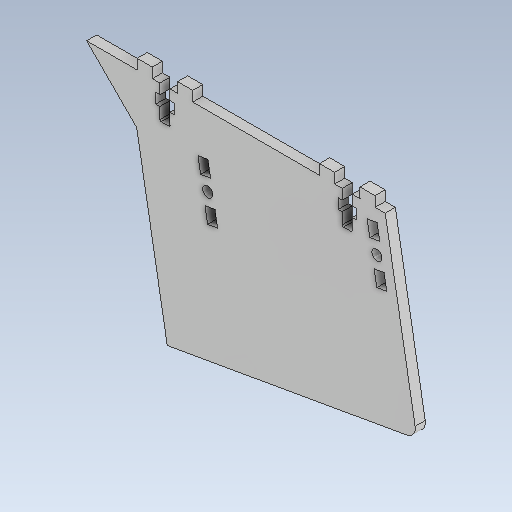
# Autodesk Inventor part: tc_support_front
Saved by Autodesk Inventor 2020.1 (Build 241239000, 239)
## iProperties
Created: 2019-07-16
Part Number: tc_support_front
Material: Acier inoxydable
Document SubType Name: Modeling
Designer: Thibault
Density: 8 g/cm^3
Appearance: Semi-poli
Author: Thibault
Autodesk Inventor part; units mm, degrees
ref_plane "YZ Plane" through (0, 0, 0) normal (1, 0, 0) x (0, 1, 0)
ref_plane "XZ Plane" through (0, 0, 0) normal (0, 1, 0) x (-1, 0, 0)
ref_plane "XY Plane" through (0, 0, 0) normal (0, 0, 1) x (1, 0, 0)
sketch "Anchor (screw side)" plane through (0, 0, 0) normal (0, 0, 1) x (1, 0, 0)
  circle A0 centre (93.7814, 50.2592) radius 1
  line L0 (91.2814, 51.2592) -> (88.2814, 51.2592)
  line L1 (88.2814, 51.2592) -> (88.2814, 49.2592)
  line L2 (88.2814, 49.2592) -> (91.2814, 49.2592)
  line L3 (91.2814, 49.2592) -> (91.2814, 51.2592)
  line L4 (99.2814, 51.2592) -> (96.2814, 51.2592)
  line L5 (96.2814, 51.2592) -> (96.2814, 49.2592)
  line L6 (96.2814, 49.2592) -> (99.2814, 49.2592)
  line L7 (99.2814, 49.2592) -> (99.2814, 51.2592)
  line L8 (91.2814, 51.2592) -> (96.2814, 49.2592) construction
  line L9 (96.2814, 51.2592) -> (91.2814, 49.2592) construction
  line L10 (86.2814, 53.2592) -> (101.2814, 53.2592) construction
  line L11 (101.2814, 53.2592) -> (101.2814, 47.2592) construction
  line L12 (101.2814, 47.2592) -> (86.2814, 47.2592) construction
  line L13 (86.2814, 47.2592) -> (86.2814, 53.2592) construction
  point P0 (103.5798, 50.1132)
  dimension "d27" = 2
  dimension "d28" = 3
  dimension "d29" = 2
  dimension "d30" = 3
  dimension "d32" = 5
  dimension "d34" = 2
  dimension "d35_1" = 2
  dimension "d36_1" = 2
  dimension "d37" = 2
  measures "d27" diameter of A0
  measures "d28" distance of L2.end L1.end
  measures "d29" distance of L1.end L0.end
  measures "d30" distance of L6.end L5.end
  measures "d32" distance between parallel lines of L5 L3
  measures "d34" distance between parallel lines of L0 L10
  measures "d35_1" distance between parallel lines of L12 L2
  measures "d36_1" distance between parallel lines of L11 L7
  measures "d37" distance between parallel lines of L13 L1
sketch "Anchor (nut side)" plane through (0, 0, 0) normal (0, 0, 1) x (1, 0, 0)
  line L0 (10, 0) -> (8.5, 0)
  line L1 (8.5, 0) -> (8.5, -2)
  line L2 (8.5, -2) -> (9.3, -2)
  line L3 (9.3, -2) -> (9.3, -4)
  line L4 (5.7, -4) -> (5.7, -2)
  line L5 (5.7, -2) -> (6.5, -2)
  line L6 (6.5, -2) -> (6.5, 0)
  line L7 (6.5, 0) -> (5, 0)
  line L8 (2, 0) -> (2, 2)
  line L9 (2, 0) -> (3, 0) construction
  line L10 (2, 2) -> (5, 2)
  line L11 (5, 2) -> (5, 0)
  line L12 (5, 2) -> (7, 2) construction
  line L13 (10, 0) -> (10, 2)
  line L14 (10, 2) -> (13, 2)
  line L15 (13, 2) -> (13, 0)
  line L16 (0, 0) -> (2, 0)
  line L17 (13, 0) -> (15, 0)
  line L18 (5.7, -4) -> (6.5, -4)
  line L19 (9.3, -4) -> (8.5, -4)
  line L20 (6.5, -4) -> (6.5, -6.25)
  line L21 (8.5, -4) -> (8.5, -6.25)
  line L22 (6.75, -6.5) -> (7.5, -6.5)
  arc A0 (6.5, -6.25) -> (6.75, -6.5) centre (6.75, -6.25) ccw
  arc A1 (8.25, -6.5) -> (8.5, -6.25) centre (8.25, -6.25) ccw
  line L23 (7.5, -7.2938) -> (7.5, -4.9797)
  line L24 (7.5, -6.5) -> (8.25, -6.5)
  point P0 (9.1321, -0.6227)
  point P1 (6.5, -6.5)
  point P2 (8.5, -6.5)
  dimension "d3" = 2
  dimension "d7" = 5
  dimension "d10" = 1.5
  dimension "d11" = 2
  dimension "d12" = 0.8
  dimension "d13" = 2
  dimension "d14" = 0.8
  dimension "d15" = 2
  dimension "d18" = 2
  dimension "d19" = 0.8
  dimension "d20" = 0.8
  dimension "d21" = 2.5
  dimension "d22" = 2.5
  dimension "d23" = 2
  dimension "d38" = 2
  dimension "d39" = 0.25
  dimension "d118" = 2
  dimension "d120" = 3
  measures "d3" distance of L16.start L8.start
  measures "d7" distance of L7.end L0.start
  measures "d10" distance of L0.start L0.end
  measures "d11" distance of L0.end L1.end
  measures "d12" distance of L1.end L2.end
  measures "d13" distance of L2.end L3.end
  measures "d14" distance of L4.end L5.end
  measures "d15" distance of L6.end L0.end
  measures "d18" distance of L15.end L17.end
  measures "d19" distance of L4.start L18.end
  measures "d20" distance of L3.end L19.end
  measures "d21" distance of L18.end point (6.5, -6.5)
  measures "d22" distance of L19.end point (8.5, -6.5)
  measures "d23" distance of L18.end L19.end
  measures "d38" distance between parallel lines of L16 L10
  measures "d39" radius of A0
  measures "d118" distance between parallel lines of L0 L14
  measures "d120" distance of L8.end L10.end
derived "shared_parameters.ipt"
sketch "Esquisse1" plane through (0, 0, 0) normal (0, 0, 1) x (1, 0, 0)
  line L0 (-2.1192, 7.2641) -> (18.9808, 7.2641)
  line L1 (-17.1192, 7.2641) -> (-25.1192, 7.2641)
  line L2 (-25.1192, 7.2641) -> (-15.2156, -2.6395)
  line L3 (39.9012, -26.3124) -> (33.9808, 7.2641)
  line L4 (38.2789, -28.6293) -> (-9.1581, -36.9937)
  line L5 (-2.0657, -1.8526) -> (7.9343, -1.7975) construction
  arc A0 (38.2789, -28.6293) -> (39.9012, -26.3124) centre (37.9316, -26.6596) ccw
  line L6 (-9.1581, -36.9937) -> (-15.2156, -2.6395)
  line L7 (-7.1192, 7.2641) -> (-8.6192, 7.2641)
  line L8 (-8.6192, 7.2641) -> (-8.6192, 5.2641)
  line L9 (-8.6192, 5.2641) -> (-7.8192, 5.2641)
  line L10 (-7.8192, 5.2641) -> (-7.8192, 3.2641)
  line L11 (-11.4192, 3.2641) -> (-11.4192, 5.2641)
  line L12 (-11.4192, 5.2641) -> (-10.6192, 5.2641)
  line L13 (-10.6192, 5.2641) -> (-10.6192, 7.2641)
  line L14 (-10.6192, 7.2641) -> (-12.1192, 7.2641)
  line L15 (-15.1192, 7.2641) -> (-15.1192, 9.2641)
  line L16 (-15.1192, 7.2641) -> (-14.1192, 7.2641) construction
  line L17 (-15.1192, 9.2641) -> (-12.1192, 9.2641)
  line L18 (-12.1192, 9.2641) -> (-12.1192, 7.2641)
  line L19 (-12.1192, 9.2641) -> (-10.1192, 9.2641) construction
  line L20 (-7.1192, 7.2641) -> (-7.1192, 9.2641)
  line L21 (-7.1192, 9.2641) -> (-4.1192, 9.2641)
  line L22 (-4.1192, 9.2641) -> (-4.1192, 7.2641)
  line L23 (-17.1192, 7.2641) -> (-15.1192, 7.2641)
  line L24 (-4.1192, 7.2641) -> (-2.1192, 7.2641)
  line L25 (-11.4192, 3.2641) -> (-10.6192, 3.2641)
  line L26 (-7.8192, 3.2641) -> (-8.6192, 3.2641)
  line L27 (-10.6192, 3.2641) -> (-10.6192, 1.0141)
  line L28 (-8.6192, 3.2641) -> (-8.6192, 1.0141)
  line L29 (-10.3692, 0.7641) -> (-9.6192, 0.7641)
  arc A1 (-10.6192, 1.0141) -> (-10.3692, 0.7641) centre (-10.3692, 1.0141) ccw
  arc A2 (-8.8692, 0.7641) -> (-8.6192, 1.0141) centre (-8.8692, 1.0141) ccw
  line L30 (-9.6192, -0.0297) -> (-9.6192, 2.2844)
  line L31 (-9.6192, 0.7641) -> (-8.8692, 0.7641)
  line L32 (28.9808, 7.2641) -> (27.4808, 7.2641)
  line L33 (27.4808, 7.2641) -> (27.4808, 5.2641)
  line L34 (27.4808, 5.2641) -> (28.2808, 5.2641)
  line L35 (28.2808, 5.2641) -> (28.2808, 3.2641)
  line L36 (24.6808, 3.2641) -> (24.6808, 5.2641)
  line L37 (24.6808, 5.2641) -> (25.4808, 5.2641)
  line L38 (25.4808, 5.2641) -> (25.4808, 7.2641)
  line L39 (25.4808, 7.2641) -> (23.9808, 7.2641)
  line L40 (20.9808, 7.2641) -> (20.9808, 9.2641)
  line L41 (20.9808, 7.2641) -> (21.9808, 7.2641) construction
  line L42 (20.9808, 9.2641) -> (23.9808, 9.2641)
  line L43 (23.9808, 9.2641) -> (23.9808, 7.2641)
  line L44 (23.9808, 9.2641) -> (25.9808, 9.2641) construction
  line L45 (28.9808, 7.2641) -> (28.9808, 9.2641)
  line L46 (28.9808, 9.2641) -> (31.9808, 9.2641)
  line L47 (31.9808, 9.2641) -> (31.9808, 7.2641)
  line L48 (18.9808, 7.2641) -> (20.9808, 7.2641)
  line L49 (31.9808, 7.2641) -> (33.9808, 7.2641)
  line L50 (24.6808, 3.2641) -> (25.4808, 3.2641)
  line L51 (28.2808, 3.2641) -> (27.4808, 3.2641)
  line L52 (25.4808, 3.2641) -> (25.4808, 1.0141)
  line L53 (27.4808, 3.2641) -> (27.4808, 1.0141)
  line L54 (25.7308, 0.7641) -> (26.4808, 0.7641)
  arc A3 (25.4808, 1.0141) -> (25.7308, 0.7641) centre (25.7308, 1.0141) ccw
  arc A4 (27.2308, 0.7641) -> (27.4808, 1.0141) centre (27.2308, 1.0141) ccw
  line L55 (26.4808, -0.0297) -> (26.4808, 2.2844)
  line L56 (26.4808, 0.7641) -> (27.2308, 0.7641)
  circle A5 centre (32.3451, -0.7359) radius 1
  line L57 (31.7944, -3.3716) -> (32.3154, -6.326)
  line L58 (32.3154, -6.326) -> (34.285, -5.9787)
  line L59 (34.285, -5.9787) -> (33.764, -3.0243)
  line L60 (33.764, -3.0243) -> (31.7944, -3.3716)
  line L61 (30.4052, 4.5069) -> (30.9262, 1.5525)
  line L62 (30.9262, 1.5525) -> (32.8958, 1.8998)
  line L63 (32.8958, 1.8998) -> (32.3748, 4.8542)
  line L64 (32.3748, 4.8542) -> (30.4052, 4.5069)
  line L65 (31.7944, -3.3716) -> (32.8958, 1.8998) construction
  line L66 (30.9262, 1.5525) -> (33.764, -3.0243) construction
  line L67 (30.693, -8.6429) -> (28.0883, 6.1292) construction
  line L68 (28.0883, 6.1292) -> (33.9972, 7.1711) construction
  line L69 (33.9972, 7.1711) -> (36.6019, -7.601) construction
  line L70 (36.6019, -7.601) -> (30.693, -8.6429) construction
  circle A6 centre (-1.1384, -6.6399) radius 1
  line L71 (-0.5877, -4.0043) -> (-1.1086, -1.0498)
  line L72 (-1.1086, -1.0498) -> (-3.0782, -1.3971)
  line L73 (-3.0782, -1.3971) -> (-2.5573, -4.3516)
  line L74 (-2.5573, -4.3516) -> (-0.5877, -4.0043)
  line L75 (0.8015, -11.8827) -> (0.2806, -8.9283)
  line L76 (0.2806, -8.9283) -> (-1.6891, -9.2756)
  line L77 (-1.6891, -9.2756) -> (-1.1681, -12.23)
  line L78 (-1.1681, -12.23) -> (0.8015, -11.8827)
  line L79 (-0.5877, -4.0043) -> (-1.6891, -9.2756) construction
  line L80 (0.2806, -8.9283) -> (-2.5573, -4.3516) construction
  line L81 (0.5137, 1.2671) -> (3.1184, -13.505) construction
  line L82 (3.1184, -13.505) -> (-2.7904, -14.5469) construction
  line L83 (-2.7904, -14.5469) -> (-5.3952, 0.2252) construction
  line L84 (-5.3952, 0.2252) -> (0.5137, 1.2671) construction
  point P0 (40.2485, -28.282)
  point P1 (22.4992, -2.0098)
  point P2 (32.3451, -0.7359)
  point P3 (-1.1384, -6.6399)
  point P4 (33.9808, 7.2641)
  dimension "d33" = 59.1
  dimension "d44" = 23
  dimension "d46" = 2
  dimension "d49" = 10
  dimension "d52" = 2
  dimension "d53" = 36
  dimension "d54" = 8
  dimension "d57" = 45
  dimension "d58" = 10
  constraints: 14 end point, 3 horizontal, 2 point on circle, 2 point on line, 2 tangent, 1 centre point, 1 parallel, 1 perpendicular, 6 other
  measures "d33" distance of L3.end L1.end
  measures "d46" radius of A0
  measures "d57" angle of L2 L1
  measures "d58" angle of L4 L0
extrude "Extrusion1" add sketch "Esquisse1" along normal blind 2
derived "tc_base_plate.ipt"
equation "\"d33\" = tc_base_width"
equation "\"d44\" = extra_height_front"
equation "\"d52\" = anchor_dist_a"
equation "\"d53\" = anchor_dist_b"
equation "\"d54\" = anchor_dist_top_a"
equation "\"d58\" = tilt_angle"
equation "\"d35\" = sheet_thickness"
equation "\"tc_base_width\" = 59.1"
equation "\"extra_height_front\" = 23"
equation "\"anchor_dist_a\" = 2"
equation "\"anchor_dist_b\" = 36"
equation "\"anchor_dist_top_a\" = 8"
equation "\"tilt_angle\" = 10deg"
equation "\"sheet_thickness\" = 2"
